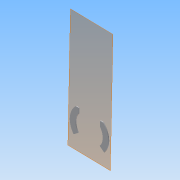
# Autodesk Inventor part: HOT Thermo bulb outline
Saved by Autodesk Inventor 2013 (Build 170138000, 138)
## iProperties
Created: 2018-07-29
Part Number: HOT Thermo bulb outline
Material: Generic
Document SubType Name: Modeling
Designer: Jeff Vyduna
Density: 1 g/cm^3
Author: Jeff Vyduna
Autodesk Inventor part; units mm, degrees
ref_plane "YZ Plane" through (0, 0, 0) normal (1, 0, 0) x (0, 1, 0)
ref_plane "XZ Plane" through (0, 0, 0) normal (0, 1, 0) x (-1, 0, 0)
ref_plane "XY Plane" through (0, 0, 0) normal (0, 0, 1) x (1, 0, 0)
ref_plane "Work Plane1" through (22.5184, 2.463, -18.3509) normal (0, 0, 1) x (0.9997722, -0.0213418, 0)
sketch "ThermoBulbBorder" plane through (22.5184, 2.463, -18.3509) normal (0, 0, 1) x (0.9997722, -0.0213418, 0)
  arc A0 (-447.455, -468.958) -> (162.145, -468.958) centre (-142.655, -774.8145) ccw
  arc A1 (-447.455, -468.958) -> (162.145, -468.958) centre (-142.655, -774.8145) ccw
  arc A2 (-383.955, -588.5959) -> (98.645, -588.5959) centre (-142.655, -774.8145) ccw
  line L0 (-447.455, -468.958) -> (-383.955, -468.958)
  line L1 (-383.955, -468.958) -> (-383.955, -588.5959)
  line L2 (162.145, -468.958) -> (98.645, -468.958)
  line L3 (98.645, -468.958) -> (98.645, -588.5959)
  line L4 (-383.955, -961.033) -> (-484.4967, -1038.6241)
  line L5 (98.645, -961.033) -> (199.1867, -1038.6241)
  arc A3 (-447.455, -468.958) -> (162.145, -468.958) centre (-142.655, -774.8145) ccw projected
  circle A4 centre (-142.655, -774.8145) radius 419.1 construction
  circle A5 centre (-142.655, -774.8145) radius 410.972 construction
  circle A6 centre (-142.655, -774.8145) radius 353.822 construction
  circle A7 centre (-142.655, -774.8145) radius 345.694 construction
  line L6 (98.645, -468.958) -> (98.645, -316.558) construction
  line L7 (-383.955, -468.958) -> (-383.955, -316.558) construction
  dimension "d0" = 609.6
  dimension "d5" = 63.5
  dimension "d6" = 63.5
  dimension "d7" = 838.2
  dimension "d8" = 8.128
  dimension "d9" = 8.128
  dimension "d10" = 57.15
  dimension "d11" = 40.894
  dimension "d12" = 152.4
  constraints: 16 end point, 12 point on circle, 7 centre point, 5 coincident, 2 concentric, 2 horizontal, 2 horizontal alignment, 2 line through centre, 2 parallel, 2 vertical, 2 vertical alignment, 1 collinear
  measures "d0" diameter of A2
  measures "d5" distance of L0.start L0.end
  measures "d6" distance of L2.start L2.end
  measures "d7" diameter of A4
  measures "d8" radial gap between concentric circles of A4 A5
  measures "d9" radial gap between concentric circles of A7 A6
  measures "d10" radial gap between concentric circles of A5 A6
  measures "d11" radial gap between concentric circles of A7 A2
  measures "d12" distance of L2.end L6.end
extrude "Sides" add sketch "ThermoBulbBorder" along normal blind 18.034 contours L0 L1 A2 L4 A0 | L5 A2 L3 L2 A0
extrude "Extrusion2" add sketch "ThermoBulbBorder" along normal blind 18.034 contours L4 A2 L5 A0
equation "\"d6\" = d5"
equation "\"d8\" = sRopeChannel"
equation "\"d9\" = sRopeChannel"
equation "\"sRopeChannel\" = 8.128"
body "Solid1"
